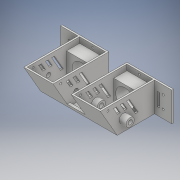
# Autodesk Inventor part: Chassi_Rear
Saved by Autodesk Inventor 2018.2 (Build 222227000, 227)
## iProperties
Created: 2018-08-12
Part Number: Chassi_Rear
Material: Generic
Document SubType Name: Modeling
Designer: mateu
Density: 1 g/cm^3
Appearance: Default
Author: mateu
Autodesk Inventor part; units mm, degrees
ref_plane "YZ Plane" through (0, 0, 0) normal (1, 0, 0) x (0, 1, 0)
ref_plane "XZ Plane" through (0, 0, 0) normal (0, 1, 0) x (-1, 0, 0)
ref_plane "XY Plane" through (0, 0, 0) normal (0, 0, 1) x (1, 0, 0)
sketch "Sketch1" plane through (0, 0, 0) normal (0, 0, 1) x (1, 0, 0)
  line L0 (0, 0) -> (110, 0)
  line L1 (110, 0) -> (110, -56)
  line L2 (110, -56) -> (0, -56)
  line L3 (0, -56) -> (0, 0)
  line L4 (0, 0) -> (-25, 0)
  line L5 (-25, 0) -> (-25, -2.4)
  line L6 (-25, -2.4) -> (0, -2.4)
  line L7 (0, -2.4) -> (0, 0)
  line L8 (110, 0) -> (135, 0)
  line L9 (135, 0) -> (135, -2.4)
  line L10 (135, -2.4) -> (110, -2.4)
  line L11 (110, -2.4) -> (110, 0)
  dimension "d0" = 110
  dimension "d1" = 56
  dimension "d2" = 25
  dimension "d3" = 2.4
  dimension "d4" = 25
  dimension "d5" = 2.4
  constraints: 24 end point, 6 parallel, 3 horizontal, 3 perpendicular
  measures "d0" distance of L1.end L2.end
  measures "d1" distance of L0.end L1.end
  measures "d2" distance of L6.end L5.end
  measures "d3" distance of L5.end L4.end
  measures "d4" distance of L9.end L10.end
  measures "d5" distance of L8.end L9.end
extrude "Extrusion1" add sketch "Sketch1" along normal blind 42
sketch "Sketch2" plane through (0, 0, 42) normal (0, 0, 1) x (1, 0, 0)
  line L0 (2.4, -2.4) -> (107.6, -2.4)
  line L1 (107.6, -2.4) -> (107.6, -54.7735)
  line L2 (2.4, -54.7735) -> (2.4, -2.4)
  line L3 (110, -56) -> (110, -2.4) projected
  line L4 (0, -2.4) -> (0, -56) projected
  line L5 (107.6, -54.7735) -> (107.6, -56)
  line L6 (2.4, -54.7735) -> (2.4, -56)
  line L7 (0, -56) -> (110, -56) projected
  point P0 (0, 0)
  dimension "d8" = 2.4
  dimension "d9" = 2.4
  constraints: 10 end point, 2 vertical, 1 horizontal, 1 parallel, 1 perpendicular, 1 point on line
  measures "d8" distance between parallel lines of L3 L1
  measures "d9" distance between parallel lines of L4 L2
extrude "Extrusion2" cut sketch "Sketch2" against normal blind 39.6
sketch "Sketch3" plane through (0, 0, 42) normal (0, 0, 1) x (1, 0, 0)
  line L0 (135, 0) -> (-25, 0) projected
  line L1 (55, 0) -> (68, 0)
  line L2 (55, 0) -> (42, 0)
  line L3 (42, 0) -> (42, -2.4)
  line L4 (2.4, -2.4) -> (107.6, -2.4) projected
  line L5 (68, -2.4) -> (42, -2.4)
  line L6 (68, -2.4) -> (68, 0)
  point P0 (0, 0)
  dimension "d12" = 13
  dimension "d13" = 13
  constraints: 10 end point, 4 point on line, 2 perpendicular, 1 collinear, 1 midpoint
  measures "d12" distance of L1.start L1.end
  measures "d13" distance of L1.start L2.end
extrude "Extrusion3" cut sketch "Sketch3" against normal blind 39.6
sketch "Sketch4" plane through (0, 0, 2.4) normal (0, 0, 1) x (1, 0, 0)
  line L0 (2.4, -2.4) -> (42, -2.4) projected
  line L1 (107.6, -56) -> (2.4, -56) projected
  line L2 (42, -2.4) -> (39.6, -2.4)
  line L3 (39.6, -2.4) -> (39.6, -56)
  line L4 (39.6, -56) -> (42, -56)
  line L5 (42, -56) -> (42, -2.4)
  line L6 (68, -2.4) -> (107.6, -2.4) projected
  line L7 (68, -2.4) -> (70.4, -2.4)
  line L8 (70.4, -2.4) -> (70.4, -56)
  line L9 (70.4, -56) -> (68, -56)
  line L10 (68, -56) -> (68, -2.4)
  point P0 (0, 0)
  dimension "d16" = 2.4
  dimension "d17" = 2.4
  constraints: 16 end point, 4 parallel, 2 horizontal, 2 perpendicular, 2 point on line
  measures "d16" distance of L4.end L3.end
  measures "d17" distance of L8.end L9.end
extrude "Extrusion4" add sketch "Sketch4" along normal blind 39.6
sketch "Sketch5" plane through (-25, -2.4, 0) normal (0, -1, 0) x (1, 0, 0)
  circle A0 centre (12.5, 30) radius 1.5
  circle A1 centre (12.5, 12) radius 1.5
  line L0 (0, 42) -> (25, 42) projected
  line L1 (0, 0) -> (25, 0) projected
  circle A2 centre (147.5, 30) radius 1.5
  circle A3 centre (147.5, 12) radius 1.5
  line L2 (0, 0) -> (0, 42) projected
  line L3 (160, 0) -> (160, 42) projected
  dimension "d20" = 3
  dimension "d21" = 3
  dimension "d22" = 12
  dimension "d23" = 12
  dimension "d51" = 3
  dimension "d52" = 3
  dimension "d53" = 12.5
  dimension "d54" = 12.5
  dimension "d55" = 12.5
  constraints: 4 centre point
  measures "d20" diameter of A0
  measures "d21" diameter of A1
  measures "d22" distance from line of L0 A0.centre
  measures "d23" distance from line of L1 A1.centre
  measures "d51" diameter of A2
  measures "d52" diameter of A3
  measures "d53" distance from line of L2 A0.centre
  measures "d54" distance from line of L3 A2.centre
  measures "d55" distance from line of L3 A3.centre
sketch "Sketch6" plane through (2.4, -2.4, 2.4) normal (0, -1, 0) x (1, 0, 0)
  line L0 (37.2, 0) -> (37.2, 39.6) projected
  line L1 (0, 39.6) -> (37.2, 39.6)
  line L2 (37.2, 39.6) -> (37.2, 0)
  line L3 (37.2, 0) -> (0, 0)
  line L4 (0, 0) -> (0, 39.6)
  line L5 (68, 39.6) -> (68, 0) projected
  line L6 (105.2, 39.6) -> (105.2, 0) projected
  line L7 (68, 39.6) -> (105.2, 39.6)
  line L8 (105.2, 39.6) -> (105.2, 0)
  line L9 (105.2, 0) -> (68, 0)
  line L10 (68, 0) -> (68, 39.6)
  point P0 (-2.4, -2.4)
  constraints: 16 end point, 4 parallel, 2 horizontal, 2 perpendicular
extrude "Extrusion5" add sketch "Sketch6" along normal blind 19
sketch "Sketch7" plane through (0, -56, 0) normal (-1, 0, 0) x (0, 0, 1)
  circle A0 centre (17, 8.6) radius 3.15
  line L0 (0, 53.6) -> (0, 0) projected
  line L1 (0, 53.6) -> (42, 53.6) projected
  point P0 (0, 56)
  dimension "d26" = 6.3
  dimension "d27" = 17
  dimension "d28" = 45
  constraints: 1 centre point
  measures "d26" diameter of A0
  measures "d27" distance from line of L0 A0.centre
  measures "d28" distance from line of L1 A0.centre
extrude "Extrusion6" cut sketch "Sketch7" against normal blind 110
sketch "Sketch8" plane through (0, -56, 0) normal (-1, 0, 0) x (0, 0, 1)
  circle A0 centre (17, 8.6) radius 3.15 projected
  circle A1 centre (17, 8.6) radius 6
  point P0 (0, 56)
  dimension "d31" = 12
  constraints: 1 centre point, 1 coincident
  measures "d31" diameter of A1
extrude "Extrusion7" add sketch "Sketch8" along normal blind 10
sketch "Sketch9" plane through (39.6, -56, 2.4) normal (-1, 0, 0) x (0, 0, 1)
  circle A0 centre (14.6, 8.6) radius 3.15 projected
  circle A1 centre (14.6, 8.6) radius 6
  point P0 (-2.4, 56)
  dimension "d34" = 12
  constraints: 1 centre point, 1 coincident
  measures "d34" diameter of A1
extrude "Extrusion8" add sketch "Sketch9" along normal blind 8
sketch "Sketch10" plane through (110, -56, 0) normal (1, 0, 0) x (0, 0, -1)
  circle A0 centre (-17, 8.6) radius 3.15 projected
  circle A1 centre (-17, 8.6) radius 6
  point P0 (0, 56)
  dimension "d37" = 12
  constraints: 1 centre point, 1 coincident
  measures "d37" diameter of A1
extrude "Extrusion9" add sketch "Sketch10" along normal blind 10
sketch "Sketch11" plane through (70.4, -56, 42) normal (1, 0, 0) x (0, 0, -1)
  circle A0 centre (25, 8.6) radius 3.15 projected
  circle A1 centre (25, 8.6) radius 6
  point P0 (42, 56)
  dimension "d40" = 12
  constraints: 1 centre point, 1 coincident
  measures "d40" diameter of A1
extrude "Extrusion10" add sketch "Sketch11" along normal blind 8
sketch "Sketch12" plane through (2.4, -21.4, 2.4) normal (0, -1, 0) x (1, 0, 0)
  circle A0 centre (21.2, 14.6) radius 13.25
  circle A1 centre (84, 14.6) radius 13.25
  line L0 (68, 0) -> (68, 39.6) projected
  line L1 (37.2, 0) -> (37.2, 39.6) projected
  line L2 (37.2, 39.6) -> (0, 39.6) projected
  line L3 (105.2, 39.6) -> (68, 39.6) projected
  point P0 (-2.4, -2.4)
  dimension "d43" = 26.5
  dimension "d44" = 26.5
  dimension "d45" = 16
  dimension "d46" = 16
  dimension "d47" = 25
  dimension "d48" = 25
  constraints: 2 centre point
  measures "d43" diameter of A0
  measures "d44" diameter of A1
  measures "d45" distance from line of L0 A1.centre
  measures "d46" distance from line of L1 A0.centre
  measures "d47" distance from line of L2 A0.centre
  measures "d48" distance from line of L3 A1.centre
extrude "Extrusion11" cut sketch "Sketch12" against normal blind 23
extrude "Extrusion12" cut sketch "Sketch5" against normal blind 20
sketch "Sketch13" plane through (-25, 0, 0) normal (0, 1, 0) x (1, 0, 0)
  line L0 (135, -11) -> (145, -11) projected
  line L1 (139.1, -30) -> (142.1, -30)
  line L2 (142.1, -30) -> (142.1, -11)
  line L3 (142.1, -11) -> (139.1, -11)
  line L4 (139.1, -11) -> (139.1, -30)
  line L5 (20.9, -30) -> (17.9, -30)
  line L6 (17.9, -30) -> (17.9, -11)
  line L7 (17.9, -11) -> (20.9, -11)
  line L8 (20.9, -11) -> (20.9, -30)
  line L9 (132.6, -42) -> (132.6, -2.4) projected
  line L10 (27.4, -2.4) -> (27.4, -42) projected
  point P0 (25, 0)
  dimension "d58" = 3
  dimension "d59" = 3
  dimension "d60" = 6.5
  dimension "d61" = 6.5
  constraints: 16 end point, 4 parallel, 3 point on line, 2 horizontal, 2 perpendicular
  measures "d58" distance of L3.end L2.end
  measures "d59" distance of L6.end L7.end
  measures "d60" distance between parallel lines of L9 L4
  measures "d61" distance between parallel lines of L10 L8
extrude "Extrusion13" cut sketch "Sketch13" against normal blind 20
sketch "Sketch21" plane through (0, -56, 0) normal (-1, 0, 0) x (0, 0, 1)
  line L0 (0, 0) -> (42, -24.2487)
  line L1 (0, 0) -> (48.4974, 0) construction
  line L2 (2.4, 0) -> (42, 0) projected
  line L3 (42, -24.2487) -> (42, 0)
  line L4 (0, 53.6) -> (0, 0) projected
  line L5 (0, 0) -> (42, 0)
  point P0 (0, 56)
  dimension "d84" = 30
  constraints: 8 end point, 2 horizontal, 1 equal length, 1 perpendicular
  measures "d84" angle of L0 L1
extrude "Extrusion21" add sketch "Sketch21" against normal blind 2.4
sketch "Sketch22" plane through (39.6, -56, 2.4) normal (-1, 0, 0) x (0, 0, 1)
  line L0 (39.6, 34.6) -> (39.6, 0) projected
  line L1 (39.6, 0) -> (-2.4, 0)
  line L2 (-2.4, 0) -> (39.6, -24.2487)
  line L3 (39.6, -24.2487) -> (39.6, 0)
  point P0 (-2.4, 56)
  dimension "d87" = 30
  constraints: 6 end point, 1 horizontal, 1 perpendicular
  measures "d87" angle of L2 L1
extrude "Extrusion22" add sketch "Sketch22" against normal blind 2.4
sketch "Sketch23" plane through (68, -56, 42) normal (-1, 0, 0) x (0, 0, 1)
  line L0 (-39.6, 0) -> (0, 0) projected
  line L1 (0, 0) -> (-42, 0)
  line L2 (-42, 0) -> (0, -24.2487)
  line L3 (0, -24.2487) -> (0, 0)
  point P0 (-42, 56)
  dimension "d90" = 30
  constraints: 6 end point, 1 horizontal, 1 perpendicular
  measures "d90" angle of L2 L1
extrude "Extrusion23" add sketch "Sketch23" against normal blind 2.4
sketch "Sketch24" plane through (107.6, -56, 2.4) normal (-1, 0, 0) x (0, 0, 1)
  line L0 (39.6, 34.6) -> (39.6, 0) projected
  line L1 (39.6, 0) -> (-2.4, 0)
  line L2 (-2.4, 0) -> (39.6, -24.2487)
  line L3 (39.6, -24.2487) -> (39.6, 0)
  point P0 (-2.4, 56)
  dimension "d93" = 30
  constraints: 6 end point, 1 horizontal, 1 perpendicular
  measures "d93" angle of L2 L1
extrude "Extrusion24" add sketch "Sketch24" against normal blind 2.4
sketch "Sketch25" plane through (107.6, -56, 2.4) normal (-1, 0, 0) x (0, 0, 1)
  line L0 (39.6, -24.2487) -> (39.6, 34.6) projected
  line L1 (-2.4, 0) -> (39.6, -24.2487)
  line L2 (39.6, -24.2487) -> (39.6, -21.8487)
  line L3 (39.6, -21.8487) -> (0, 0)
  line L4 (-2.4, 0) -> (0, 0) projected
  line L5 (0, 0) -> (-2.4, 0)
  point P0 (-2.4, 56)
  dimension "d96" = 2.4
  constraints: 8 end point, 1 collinear, 1 point on line
  measures "d96" distance of L0.start L2.end
extrude "Extrusion25" add sketch "Sketch25" along normal blind 38
sketch "Sketch26" plane through (2.4, -56, 2.4) normal (1, 0, 0) x (0, 0, -1)
  line L0 (2.4, 53.6) -> (2.4, 0) projected
  line L1 (0, 0) -> (2.4, 0)
  line L2 (-39.6, -24.2487) -> (2.4, 0) projected
  line L3 (2.4, 0) -> (-39.6, -24.2487)
  line L4 (-39.6, -24.2487) -> (-39.6, -21.8487)
  line L5 (-39.6, 34.6) -> (-39.6, -24.2487) projected
  line L6 (-39.6, -21.8487) -> (0, 0)
  point P0 (2.4, 56)
  dimension "d99" = 2.4
  constraints: 8 end point, 1 collinear, 1 horizontal, 1 point on line
  measures "d99" distance of L2.start L4.end
extrude "Extrusion26" add sketch "Sketch26" along normal blind 38
sketch "Sketch27" plane through (42, -56, 2.4) normal (1, 0, 0) x (0, 0, -1)
  line L0 (0, 0) -> (2.4, 0) projected
  line L1 (2.4, 0) -> (-4.6, 0)
  line L2 (-4.6, 0) -> (-4.6, -4.0415)
  line L3 (-39.6, -24.2487) -> (2.4, 0) projected
  line L4 (-4.6, -4.0415) -> (2.4, 0)
  point P0 (2.4, 56)
  dimension "d102" = 7
  dimension "d103" = 90
  constraints: 6 end point, 1 collinear, 1 point on line
  measures "d102" distance of L0.end L1.end
  measures "d103" angle of L2 L1
extrude "Extrusion27" add sketch "Sketch27" along normal blind 26
sketch "Sketch28" plane through (0, -2.4, 0) normal (-1, 0, 0) x (0, 0, 1)
  circle A0 centre (37, -66.8791) radius 1.5
  line L0 (42, 0) -> (42, -77.8487) projected
  line L1 (0, -53.6) -> (42, -77.8487) projected
  point P0 (0, 2.4)
  dimension "d106" = 3
  dimension "d107" = 5
  dimension "d108" = 7
  constraints: 1 centre point
  measures "d106" diameter of A0
  measures "d107" distance from line of L0 A0.centre
  measures "d108" distance from line of L1 A0.centre
extrude "Extrusion28" cut sketch "Sketch28" against normal blind 120
sketch "Sketch29" plane through (110, -2.4, 42) normal (1, 0, 0) x (0, 0, -1)
  line L0 (6, -59.0216) -> (16, -53.2481)
  line L1 (0, -77.8487) -> (42, -53.6) projected
  line L2 (6, -59.0216) -> (6, -55.0216)
  line L3 (6, -55.0216) -> (16, -49.2481)
  line L4 (16, -49.2481) -> (16, -53.2481)
  line L5 (6, -49.2481) -> (6, -45.2481)
  line L6 (6, -45.2481) -> (16, -39.4746)
  line L7 (16, -39.4746) -> (16, -43.4746)
  line L8 (16, -43.4746) -> (6, -49.2481)
  line L9 (0, 0) -> (0, -77.8487) projected
  line L10 (6, -40.2481) -> (6, -36.2481)
  line L11 (6, -36.2481) -> (27.9337, -23.5847)
  line L12 (27.9337, -23.5847) -> (27.9337, -27.5847)
  line L13 (27.9337, -27.5847) -> (6, -40.2481)
  point P0 (42, 2.4)
  dimension "d111" = 4
  dimension "d112" = 10
  dimension "d113" = 4
  dimension "d114" = 4
  dimension "d115" = 10
  dimension "d116" = 6
  dimension "d117" = 6
  dimension "d118" = 5
  dimension "d119" = 4
  dimension "d120" = 4
  dimension "d121" = 5
  dimension "d122" = 6
  constraints: 24 end point, 7 parallel, 3 vertical
  measures "d111" distance of L0.start L2.end
  measures "d112" horizontal distance of L0.start L0.end
  measures "d113" distance of L5.start L5.end
  measures "d114" distance of L6.end L7.end
  measures "d115" horizontal distance of L7.end L5.start
  measures "d116" distance between parallel lines of L9 L2
  measures "d117" distance between parallel lines of L9 L5
  measures "d118" distance between parallel lines of L3 L8
  measures "d119" distance of L10.start L10.end
  measures "d120" distance of L11.end L12.end
  measures "d121" distance of L10.start L5.end
  measures "d122" distance between parallel lines of L9 L10
extrude "Extrusion29" cut sketch "Sketch29" against normal blind 120
sketch "Sketch31" plane through (0, 0, 42) normal (0, 0, 1) x (1, 0, 0)
  line L0 (39.6, -21.4) -> (39.6, -77.8487) projected
  line L1 (2.4, -2.4613) -> (39.6, -2.4613)
  line L2 (39.6, -2.4613) -> (39.6, -21.4)
  line L3 (39.6, -21.4) -> (2.4, -21.4)
  line L4 (2.4, -21.4) -> (2.4, -2.4613)
  line L5 (70.4, -21.4) -> (70.4, -77.8487) projected
  line L6 (70.4, -21.4) -> (107.6193, -21.4)
  line L7 (107.6193, -21.4) -> (107.6193, -2.4613)
  line L8 (107.6193, -2.4613) -> (70.4, -2.4613)
  line L9 (70.4, -2.4613) -> (70.4, -21.4)
  point P0 (0, 0)
  constraints: 16 end point, 4 parallel, 2 horizontal, 2 perpendicular, 1 point on line
extrude "Extrusion30" cut sketch "Sketch31" against normal blind 8
sketch "Sketch32" plane through (2.4, -2.4613, 42) normal (0, -1, 0) x (1, 0, 0)
  circle A0 centre (19.2, -4) radius 1.5
  circle A1 centre (86, -4) radius 1.5
  line L0 (0, 0) -> (37.2, 0) projected
  line L1 (68, 0) -> (105.2193, 0) projected
  point P0 (-2.4, -42)
  dimension "d127" = 3
  dimension "d128" = 3
  dimension "d129" = 4
  dimension "d130" = 4
  dimension "d131" = 18
  dimension "d132" = 18
  constraints: 2 centre point
  measures "d127" diameter of A0
  measures "d128" diameter of A1
  measures "d129" distance from line of L0 A0.centre
  measures "d130" distance from line of L1 A1.centre
  measures "d131" horizontal distance of L1.start A1.centre
  measures "d132" horizontal distance of L0.end A0.centre
extrude "Extrusion31" cut sketch "Sketch32" against normal blind 8
equation "\"d54\" = d53"
equation "\"d55\" = d54"
body "Solid1"
